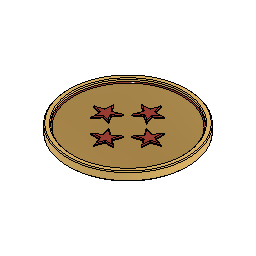
Dragon Ball v1 (Autodesk Fusion 360 design; units mm, degrees)
Autodesk Fusion 360 part; units mm, degrees
sketch "Sketch1" plane through (0, 0, 0) normal (0, 0, 1) x (1, 0, 0)
sketch "Sketch2" plane through (0, 0, 0) normal (0, 0, 1) x (1, 0, 0)
  circle A0 centre (0, 0) radius 8.752
  circle A1 centre (0, 0) radius 8.0085
  line L0 (-0.4742, 3.7643) -> (-0.0652, 4.9615)
  line L1 (-0.0652, 4.9615) -> (0.3439, 3.7643)
  line L2 (0.3439, 3.7643) -> (-0.4742, 3.7643) construction
  line L3 (-0.0652, 4.9615) -> (-0.0652, 3.7643) construction
  line L4 (-0.4742, 3.7643) -> (-0.0652, 3.1545) construction
  line L5 (-0.0652, 3.1545) -> (-0.0652, 3.7643) construction
  line L6 (-0.0652, 3.1545) -> (0.3439, 3.7643) construction
  line L7 (-0.0652, 3.1545) -> (-0.0652, 0) construction
  line L8 (-0.0652, 0) -> (0, 0) construction
  line L9 (-0.7715, 2.9539) -> (-1.7837, 3.7129)
  line L10 (-1.7837, 3.7129) -> (-0.5187, 3.732)
  line L11 (-0.0927, 2.4208) -> (-1.1273, 1.6927)
  line L12 (-1.1273, 1.6927) -> (-0.7545, 2.9016)
  line L13 (0.6242, 2.9016) -> (0.9969, 1.6927)
  line L14 (0.9969, 1.6927) -> (-0.0377, 2.4208)
  line L15 (0.3883, 3.732) -> (1.6533, 3.7129)
  line L16 (1.6533, 3.7129) -> (0.6411, 2.9539)
  line L17 (0.3439, 3.7643) -> (0.3883, 3.732)
  line L18 (0.6411, 2.9539) -> (0.6242, 2.9016)
  line L19 (-0.0927, 2.4208) -> (-0.0377, 2.4208)
  line L20 (-0.7715, 2.9539) -> (-0.7545, 2.9016)
  line L21 (-0.4742, 3.7643) -> (-0.5187, 3.732)
  line L22 (-3.7781, -1.7185) -> (-3.7971, -0.4535)
  line L23 (-3.8295, -0.409) -> (-5.0267, 0)
  line L24 (-3.8295, -0.409) -> (-3.7971, -0.4535)
  line L25 (-3.0191, -0.7063) -> (-3.7781, -1.7185)
  line L26 (-3.0191, -0.7063) -> (-2.9668, -0.6893)
  line L27 (-1.7578, -1.0621) -> (-2.9668, -0.6893)
  line L28 (-5.0267, 0) -> (-3.8295, 0.409)
  line L29 (-3.8295, 0.409) -> (-3.7971, 0.4535)
  line L30 (-3.7971, 0.4535) -> (-3.7781, 1.7185)
  line L31 (-3.7781, 1.7185) -> (-3.0191, 0.7063)
  line L32 (-3.0191, 0.7063) -> (-2.9668, 0.6893)
  line L33 (-2.9668, 0.6893) -> (-1.7578, 1.0621)
  line L34 (-1.7578, 1.0621) -> (-2.486, 0.0275)
  line L35 (-2.486, -0.0275) -> (-1.7578, -1.0621)
  line L36 (-2.486, -0.0275) -> (-2.486, 0.0275)
  line L37 (1.6533, -3.7129) -> (0.3883, -3.732)
  line L38 (0.3439, -3.7643) -> (-0.0652, -4.9615)
  line L39 (0.3439, -3.7643) -> (0.3883, -3.732)
  line L40 (0.6411, -2.9539) -> (1.6533, -3.7129)
  line L41 (0.6411, -2.9539) -> (0.6242, -2.9016)
  line L42 (0.9969, -1.6927) -> (0.6242, -2.9016)
  line L43 (-0.0652, -4.9615) -> (-0.4742, -3.7643)
  line L44 (-0.4742, -3.7643) -> (-0.5187, -3.732)
  line L45 (-0.5187, -3.732) -> (-1.7837, -3.7129)
  line L46 (-1.7837, -3.7129) -> (-0.7715, -2.9539)
  line L47 (-0.7715, -2.9539) -> (-0.7545, -2.9016)
  line L48 (-0.7545, -2.9016) -> (-1.1273, -1.6927)
  line L49 (-1.1273, -1.6927) -> (-0.0927, -2.4208)
  line L50 (-0.0377, -2.4208) -> (0.9969, -1.6927)
  line L51 (-0.0377, -2.4208) -> (-0.0927, -2.4208)
  line L52 (3.6477, 1.7185) -> (3.6668, 0.4535)
  line L53 (3.6991, 0.409) -> (4.8963, 0)
  line L54 (3.6991, 0.409) -> (3.6668, 0.4535)
  line L55 (2.8887, 0.7063) -> (3.6477, 1.7185)
  line L56 (2.8887, 0.7063) -> (2.8364, 0.6893)
  line L57 (1.6275, 1.0621) -> (2.8364, 0.6893)
  line L58 (4.8963, 0) -> (3.6991, -0.409)
  line L59 (3.6991, -0.409) -> (3.6668, -0.4535)
  line L60 (3.6668, -0.4535) -> (3.6477, -1.7185)
  line L61 (3.6477, -1.7185) -> (2.8887, -0.7063)
  line L62 (2.8887, -0.7063) -> (2.8364, -0.6893)
  line L63 (2.8364, -0.6893) -> (1.6275, -1.0621)
  line L64 (1.6275, -1.0621) -> (2.3556, -0.0275)
  line L65 (2.3556, 0.0275) -> (1.6275, 1.0621)
  line L66 (2.3556, 0.0275) -> (2.3556, -0.0275)
  dimension "d1" = 17.5041
  dimension "d2" = 0.0652
  dimension "d3" = 3.1545
  dimension "d4" = 0.7343
  dimension "d5" = 0.6098
  dimension "d6" = 1.1972
  dimension "d8" = 360
  dimension "d10" = 360
  constraint coincident A0.centre A1.centre
  constraint horizontal L2
  constraint equal L0 L1
  constraint midpoint L2 L3.end
  constraint perpendicular L2 L3
  constraint perpendicular L2 L5
  constraint parallel L5 L7
  constraint perpendicular L5 L8
  constraint perpendicular L7 L19
  measures "d1" diameter of A0
  measures "d2" distance of L7.end A0.centre
  measures "d3" distance of L4.end L7.end
  measures "d4" distance of L1.end L4.end
  measures "d5" distance of L3.end L4.end
  measures "d6" distance of L0.end L3.end
extrude "Extrude1" add sketch "Sketch2" along normal blind 1.27 contours A0 | A1 | L0 L1 L9 L10 L11 L12 L13 L14 L15 L16 L17 L18 L19 L20 L21 | L22 L23 L24 L25 L26 L27 L28 L29 L30 L31 L32 L33 L34 L35 L36 | L37 L38 L39 L40 L41 L42 L43 L44 L45 L46 L47 L48 L49 L50 L51 | L52 L53 L54 L55 L56 L57 L58 L59 L60 L61 L62 L63 L64 L65 L66
sketch "Sketch4" plane through (0, 0, 1.27) normal (0, 0, 1) x (-1, 0, 0)
  circle A0 centre (0, 0) radius 8.752
  circle A1 centre (0, 0) radius 8.0085
extrude "Extrude2" cut sketch "Sketch4" against normal blind 0.508 contours A1
sketch "Sketch5" plane through (0, 0, 0.762) normal (0, 0, 1) x (-1, 0, 0)
  circle A0 centre (0, 0) radius 8.0085
  line L0 (-1.6533, -3.7129) -> (-0.6411, -2.9539)
  line L1 (-0.3883, -3.732) -> (-1.6533, -3.7129)
  line L2 (0.0652, -4.9615) -> (-0.3439, -3.7643)
  line L3 (0.4742, -3.7643) -> (0.0652, -4.9615)
  line L4 (1.7837, -3.7129) -> (0.5187, -3.732)
  line L5 (0.7715, -2.9539) -> (1.7837, -3.7129)
  line L6 (-0.3439, -3.7643) -> (-0.3883, -3.732)
  line L7 (0.4742, -3.7643) -> (0.5187, -3.732)
  line L8 (0.7715, -2.9539) -> (0.7545, -2.9016)
  line L9 (1.1273, -1.6927) -> (0.7545, -2.9016)
  line L10 (0.0927, -2.4208) -> (1.1273, -1.6927)
  line L11 (0.0927, -2.4208) -> (0.0377, -2.4208)
  line L12 (-0.9969, -1.6927) -> (0.0377, -2.4208)
  line L13 (-0.6242, -2.9016) -> (-0.9969, -1.6927)
  line L14 (-0.6411, -2.9539) -> (-0.6242, -2.9016)
  line L15 (-2.8887, -0.7063) -> (-3.6477, -1.7185)
  line L16 (-3.6477, -1.7185) -> (-3.6668, -0.4535)
  line L17 (-1.6275, -1.0621) -> (-2.8364, -0.6893)
  line L18 (-2.3556, -0.0275) -> (-1.6275, -1.0621)
  line L19 (-2.8887, -0.7063) -> (-2.8364, -0.6893)
  line L20 (-3.6991, -0.409) -> (-3.6668, -0.4535)
  line L21 (-3.6991, -0.409) -> (-4.8963, 0)
  line L22 (-4.8963, 0) -> (-3.6991, 0.409)
  line L23 (-3.6991, 0.409) -> (-3.6668, 0.4535)
  line L24 (-3.6668, 0.4535) -> (-3.6477, 1.7185)
  line L25 (-3.6477, 1.7185) -> (-2.8887, 0.7063)
  line L26 (-2.8887, 0.7063) -> (-2.8364, 0.6893)
  line L27 (-2.8364, 0.6893) -> (-1.6275, 1.0621)
  line L28 (-1.6275, 1.0621) -> (-2.3556, 0.0275)
  line L29 (-2.3556, -0.0275) -> (-2.3556, 0.0275)
  line L30 (0.7545, 2.9016) -> (1.1273, 1.6927)
  line L31 (1.1273, 1.6927) -> (0.0927, 2.4208)
  line L32 (0.0377, 2.4208) -> (0.0927, 2.4208)
  line L33 (0.0377, 2.4208) -> (-0.9969, 1.6927)
  line L34 (-0.9969, 1.6927) -> (-0.6242, 2.9016)
  line L35 (-0.6411, 2.9539) -> (-0.6242, 2.9016)
  line L36 (-0.6411, 2.9539) -> (-1.6533, 3.7129)
  line L37 (-1.6533, 3.7129) -> (-0.3883, 3.732)
  line L38 (-0.3439, 3.7643) -> (-0.3883, 3.732)
  line L39 (-0.3439, 3.7643) -> (0.0652, 4.9615)
  line L40 (0.0652, 4.9615) -> (0.4742, 3.7643)
  line L41 (0.4742, 3.7643) -> (0.5187, 3.732)
  line L42 (0.5187, 3.732) -> (1.7837, 3.7129)
  line L43 (1.7837, 3.7129) -> (0.7715, 2.9539)
  line L44 (0.7715, 2.9539) -> (0.7545, 2.9016)
  line L45 (5.0267, 0) -> (3.8295, -0.409)
  line L46 (3.7971, -0.4535) -> (3.7781, -1.7185)
  line L47 (3.7781, -1.7185) -> (3.0191, -0.7063)
  line L48 (2.9668, -0.6893) -> (1.7578, -1.0621)
  line L49 (3.8295, -0.409) -> (3.7971, -0.4535)
  line L50 (3.0191, -0.7063) -> (2.9668, -0.6893)
  line L51 (1.7578, -1.0621) -> (2.486, -0.0275)
  line L52 (2.486, 0.0275) -> (1.7578, 1.0621)
  line L53 (2.486, 0.0275) -> (2.486, -0.0275)
  line L54 (1.7578, 1.0621) -> (2.9668, 0.6893)
  line L55 (3.0191, 0.7063) -> (2.9668, 0.6893)
  line L56 (3.0191, 0.7063) -> (3.7781, 1.7185)
  line L57 (3.8295, 0.409) -> (5.0267, 0)
  line L58 (3.8295, 0.409) -> (3.7971, 0.4535)
  line L59 (3.7781, 1.7185) -> (3.7971, 0.4535)
extrude "Extrude3" add sketch "Sketch5" along normal blind 0.254 contours L0 L1 L2 L3 L4 L5 L6 L7 L8 L9 L10 L11 L12 L13 L14 | L15 L16 L17 L18 L19 L20 L21 L22 L23 L24 L25 L26 L27 L28 L29 | L30 L31 L32 L33 L34 L35 L36 L37 L38 L39 L40 L41 L42 L43 L44 | L45 L46 L47 L48 L49 L50 L51 L52 L53 L54 L55 L56 L57 L58 L59
fillet "Fillet1" radius 0.127 1 edges at (7.4665, -2.896, 0.762)
fillet "Fillet2" radius 0.127 3 edges at (7.4665, -2.896, 1.27) (-8.1598, -3.1649, 1.27) (-8.1598, -3.1649, 0)
fillet "Fillet3" radius 0.127 1 faces at (0.0917, 3.1958, 1.016)
fillet "Fillet4" radius 0.127 1 faces at (3.1481, 0.1512, 1.016)
fillet "Fillet5" radius 0.127 1 faces at (-0.222, -3.1958, 1.016)
fillet "Fillet6" radius 0.127 1 faces at (-3.2785, 0.1512, 1.016)
